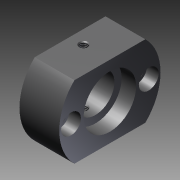
# Autodesk Inventor part: BGCSB9_h
Saved by Autodesk Inventor 2016 (Build 200138000, 138)
## iProperties
Category: PARTsolutions
Company: MISUMI
Created: 2016-11-09
Part Number: BGCSB9_h
Catalog Web Link: www.cadenas.de
Description: BGCSB, BGCS, SBGCS_housing-Bearing with Housings - Thrust Bearings - Standard
Vendor: MISUMI
Document SubType Name: Modeling
Designer: psAdmin
Manufacturer: MISUMI
Mass: 31.9645 g
Surface Area: 98.222 cm^2
Volume: 31.9645 cm^3
Density: 1 g/cm^3
Material: 一般
Appearance: PSOLRGB-192-192-192
PSOL_IDENT_0: {$CADENAS_DATA\23d-libs\misumi\metric\12_bearing_holders\bgcsb\housing_bgcsb.prj},182 {VTYP=3D},{NB=
PSOL_IDENT_1: BGCSB9_h},{LINA=BGCSB9},{NN=BGCSB, BGCS, SBGCS_housing},{DATE=17.06.2016 05:47:01},{GEOMDATE=02.03.2
PSOL_IDENT_2: 016 00:34:00},{VERSION=},{LINEID=20},{LINESUBID=-1},{WBVAR=MAT,ST}  {NB=BGCSB9_h},{LINA=BGCSB9},{KT=
PSOL_IDENT_3: DUMMY},{PN=BGCSB9},{TYPE=BGCSB},{MAT=BG},{MAT1= 'BG','S45C Equivalent','SBG','SUS304' },{ST=B},{ST1=
PSOL_IDENT_4: 'B','Black Oxide','ENP','Electroless Nickel Plating'               },{DD=9},{D=21},{B=23},{H=56}
PSOL_IDENT_5: ,{W=40},{T=22},{DDZZ=12},{D1=27},{D2=29},{D3=26},{T1=14},{B1=15.5},{A=43},{F=0},{M=M8 (6.8)},{DD1=11
PSOL_IDENT_6: },{H1=6.5},{BN=NKXZ9},{DD2=6.800},{MMAX=8.000},{M1=5},{M1L=9.5}
NN: BGCSB, BGCS, SBGCS_housing
NT: Bearing with Housings - Thrust Bearings - Standard
NB: BGCSB9_h
NBSYN: $PN._h
LINA: BGCSB9
PN: BGCSB9
MAT: S45C Equivalent
ST: Black Oxide
DD: 9
D: 21
B: 23
H: 56
W: 40
T: 22
DDZZ: 12
D1: 27
D2: 29
D3: 26
T1: 14
B1: 15.5
A: 43
F: 0
M: M8 (6.8)
DD1: 11
H1: 6.5
BN: NKXZ9
SUPPLIER: MISUMI
ARTICLENO: BGCSB9_h
BOMINFO: BGCSB9
CREATOR: CADENAS GmbH
Title: BGCSB9
Author: Cadenas PARTsolutions
Comments: Bearing with Housings - Thrust Bearings - Standard
Autodesk Inventor part; units mm, degrees
sketch "Sketch_1" plane through (0, 0, 0) normal (0, 0, 1) x (1, 0, 0)
  line L0 (22, 0) -> (0, 0)
  line L1 (0, 28) -> (0, 10.5)
  line L2 (0, 10.5) -> (14, 10.5)
  line L3 (14, 10.5) -> (14, 14.5)
  line L4 (14, 14.5) -> (22, 14.5)
  line L5 (22, 14.5) -> (22, 28)
  line L6 (22, 28) -> (0, 28)
  constraints: 14 end point
revolve "Revolution1" add sketch "Sketch_1" angle 360 about axis through (22, 0, 0) along (1, 0, 0)
sketch "Sketch_2" plane through (0, 0, 0) normal (1, 0, 0) x (0, 1, 0)
  line L0 (-112, 80) -> (-112, -80)
  line L1 (-112, -80) -> (112, -80)
  line L2 (112, -80) -> (112, 80)
  line L3 (112, 80) -> (-112, 80)
  line L4 (-28, 20) -> (-28, -20)
  line L5 (-28, -20) -> (28, -20)
  line L6 (28, -20) -> (28, 20)
  line L7 (28, 20) -> (-28, 20)
  constraints: 16 end point
extrude "Extrusion1" cut sketch "Sketch_2" along normal blind 24
sketch "Sketch_3" plane through (0, 0, 0) normal (0, 0, 1) x (1, 0, 0)
  line L0 (22, 21.5) -> (0, 21.5)
  line L1 (0, 21.5) -> (0, 25.5)
  line L2 (0, 25.5) -> (0.6765, 24.8235)
  line L3 (0.6765, 24.8235) -> (14.8235, 24.8235)
  line L4 (14.8235, 24.8235) -> (15.5, 25.5)
  line L5 (15.5, 25.5) -> (15.5, 27)
  line L6 (15.5, 27) -> (22, 27)
  line L7 (22, 27) -> (22, 21.5)
  line L8 (22, 21.5) -> (0, 21.5)
  constraints: 18 end point
revolve "Revolution2" cut sketch "Sketch_3" angle 360 about axis through (22, 21.5, 0) along (1, 0, 0)
thread "Thread1" size "M8x1.25" class "6H" standard "ISO Metric profile" full length
pattern_linear "Rectangular Pattern1" count 2 spacing 43 along (0, -1, 0) of "Revolution2"
sketch "Sketch_4" plane through (7.5, 0, 0) normal (1, 0, 0) x (0, 0, -1)
  line L0 (-10.15, 0) -> (-20, 0)
  line L1 (-20, 0) -> (-20, 2.5)
  line L2 (-20, 2.5) -> (-19.567, 2.067)
  line L3 (-19.567, 2.067) -> (-10.583, 2.067)
  line L4 (-10.583, 2.067) -> (-10.15, 2.5)
  line L5 (-10.15, 2.5) -> (-10.15, 0)
  line L6 (-10.15, 0) -> (-20, 0)
  constraints: 14 end point
revolve "Revolution3" cut sketch "Sketch_4" angle 360 about axis through (7.5, 0, 10.15) along (0, 0, -1)
thread "Thread2" size "M5x0.8" class "6H" standard "ISO Metric profile" full length
sketch "Sketch_6" plane through (7.5, 0, 0) normal (1, 0, 0) x (0, 0, -1)
  line L0 (20, 0) -> (10.15, 0)
  line L1 (10.15, 0) -> (10.15, 2.5)
  line L2 (10.15, 2.5) -> (10.583, 2.067)
  line L3 (10.583, 2.067) -> (19.567, 2.067)
  line L4 (19.567, 2.067) -> (20, 2.5)
  line L5 (20, 2.5) -> (20, 0)
  line L6 (20, 0) -> (10.15, 0)
  constraints: 14 end point
revolve "Revolution4" cut sketch "Sketch_6" angle 360 about axis through (7.5, 0, -20) along (0, 0, -1)
thread "Thread3" size "M5x0.8" class "6H" standard "ISO Metric profile" full length
ref_plane "to_bearings_XY" through (14, 0, 0) normal (1, 0, 0) x (0, 0, -1)
ref_plane "to_bearings_YZ" through (14, 0, 0) normal (0, 0, -1) x (0, 1, 0)
ref_plane "to_bearings_ZX" through (14, 0, 0) normal (0, 1, 0) x (1, 0, 0)
ref_plane "to_screw1_XY" through (7.5, 0, 10.5) normal (0, 0, 1) x (1, 0, 0)
ref_plane "to_screw1_YZ" through (7.5, 0, 10.5) normal (1, 0, 0) x (0, 1, 0)
ref_plane "to_screw1_ZX" through (7.5, 0, 10.5) normal (0, 1, 0) x (0, 0, 1)
ref_plane "to_screw2_XY" through (7.5, 0, -10.5) normal (0, 0, -1) x (1, 0, 0)
ref_plane "to_screw2_YZ" through (7.5, 0, -10.5) normal (1, 0, 0) x (0, -1, 0)
ref_plane "to_screw2_ZX" through (7.5, 0, -10.5) normal (0, -1, 0) x (0, 0, -1)
body "Solid1"
